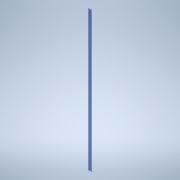
# Autodesk Inventor part: SP54V1 Acrilico inferior
Saved by Autodesk Inventor 2021.2 (Build 252289000, 289)
## iProperties
Created: 2026-09-28
Part Number: SP54V1 Acrilico inferior
Material: Polycarbonate, Clear
Document SubType Name: Modeling
Designer: nelso
Density: 1.2 g/cm^3
Appearance: Clear - Blue
Author: nelso
Autodesk Inventor part; units mm, degrees
ref_plane "YZ Plane" through (0, 0, 0) normal (1, 0, 0) x (0, 1, 0)
ref_plane "XZ Plane" through (0, 0, 0) normal (0, 1, 0) x (-1, 0, 0)
ref_plane "XY Plane" through (0, 0, 0) normal (0, 0, 1) x (1, 0, 0)
sketch "Sketch1" plane through (0, 0, 0) normal (0, 1, 0) x (-1, 0, 0)
  line L0 (-20, 825) -> (20, 825)
  line L1 (20, 825) -> (20, -825)
  line L2 (20, -825) -> (-20, -825)
  line L3 (-20, -825) -> (-20, 825)
  line L4 (-20, 825) -> (20, -825) construction
  line L5 (20, 825) -> (-20, -825) construction
  point P0 (0, 0)
  dimension "d0" = 40
  dimension "d1" = 1650
  constraints: 12 end point, 2 midpoint, 2 parallel, 1 horizontal, 1 perpendicular
  measures "d0" distance of L1.end L2.end
  measures "d1" distance of L0.end L1.end
extrude "Extrusion1" add sketch "Sketch1" along normal blind 3
sketch "Sketch2" plane through (0, 3, 0) normal (0, 1, 0) x (1, 0, 0)
  line L0 (20, 825) -> (-20, 825) projected
  line L1 (0, 825) -> (0, 815)
  line L2 (0, 815) -> (-10, 815)
  point P0 (0, 0)
  point P1 (10, 815)
  point P2 (10, 815)
  dimension "d4" = 10
  dimension "d5" = 10
  constraints: 4 end point, 2 coincident, 2 symmetric about line, 1 midpoint, 1 perpendicular, 1 vertical
  measures "d4" distance of L1.start L1.end
  measures "d5" distance of L1.end L2.end
hole "Hole1" at (-10, 3, -815) at (10, 3, -815) direction (0, -1, 0) diameter 4.5 depth 8 clearance for "Countersunk Flat Head Screw ISO 2009/7046" size "M4" standard "ISO"
body "Solid1"
